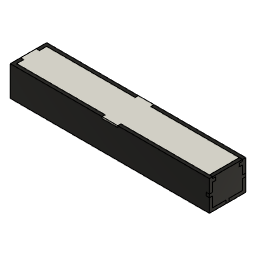
Soporte_LEDs v2 (Autodesk Fusion 360 design; units mm, degrees)
Autodesk Fusion 360 part; units mm, degrees
sketch "Boceto1" plane through (0, 0, 0) normal (0, 0, 1) x (1, 0, 0)
  line L0 (60, 8.75) -> (-60, 8.75)
  line L1 (-60, 8.75) -> (-60, -8.75)
  line L2 (-60, -8.75) -> (60, -8.75)
  line L3 (60, -8.75) -> (60, 8.75)
  line L4 (60, 8.75) -> (-60, -8.75) construction
  line L5 (-60, 8.75) -> (60, -8.75) construction
  dimension "d1" = 120
  dimension "d2" = 17.5
  constraint horizontal L0
  constraint perpendicular L0 L1
  constraint parallel L0 L2
  constraint parallel L1 L3
  constraint coincident L4 origin
  constraint coincident L5 origin
  measures "d1" distance of L1.end L2.end
  measures "d2" distance of L0.end L1.end
sketch "Boceto2" plane through (0, 0, 0) normal (0, 0, 1) x (1, 0, 0)
  line L0 (62, 9.5) -> (-62, 9.5)
  line L1 (-62, 9.5) -> (-62, -9.5)
  line L2 (-62, -9.5) -> (62, -9.5)
  line L3 (62, -9.5) -> (62, 9.5)
  line L4 (62, 9.5) -> (-62, -9.5) construction
  line L5 (-62, 9.5) -> (62, -9.5) construction
  line L6 (64, 11.5) -> (-64, 11.5)
  line L7 (-64, 11.5) -> (-64, -11.5)
  line L8 (-64, -11.5) -> (64, -11.5)
  line L9 (64, -11.5) -> (64, 11.5)
  line L10 (64, 11.5) -> (-64, -11.5) construction
  line L11 (-64, 11.5) -> (64, -11.5) construction
  dimension "d3" = 124
  dimension "d4" = 19
  dimension "d5" = 128
  dimension "d6" = 23
  constraint horizontal L0
  constraint perpendicular L0 L1
  constraint parallel L0 L2
  constraint parallel L1 L3
  constraint coincident L4 origin
  constraint coincident L5 origin
  constraint horizontal L6
  constraint perpendicular L6 L7
  constraint parallel L6 L8
  constraint parallel L7 L9
  constraint coincident L10 origin
  constraint coincident L11 origin
  measures "d3" distance of L1.end L2.end
  measures "d4" distance of L0.end L1.end
  measures "d5" distance of L7.end L8.end
  measures "d6" distance of L6.end L7.end
extrude "Extruir1" add sketch "Boceto2" along normal blind 2 contours L0 L1 L2 L3 makes body 1
extrude "Extruir2" add sketch "Boceto2" along normal blind 19 bodies 1
extrude "Extruir3" cut 1 faces at (64, -3.8333, 12.6667) along direction (-1, 0, 0) blind 2 on bodies 1 bodies 1
sketch "Boceto3" plane through (62, 0, 0) normal (1, 0, 0) x (0, 1, 0)
  line L0 (9.5, 19) -> (9.5, 2)
  line L1 (9.5, 2) -> (-9.5, 2)
  line L2 (-9.5, 2) -> (-9.5, 19)
  line L3 (-9.5, 19) -> (-11.5, 19)
  line L4 (-11.5, 19) -> (-11.5, 0)
  line L5 (-11.5, 0) -> (11.5, 0)
  line L6 (11.5, 0) -> (11.5, 19)
  line L7 (11.5, 19) -> (9.5, 19)
  line L8 (-11.5, 19) -> (11.5, 19)
  line L9 (11.5, 19) -> (11.5, 0)
  line L10 (11.5, 0) -> (-11.5, 0)
  line L11 (-11.5, 0) -> (-11.5, 19)
  line L12 (-11.5, 19) -> (-9.5, 19)
  line L13 (-9.5, 2) -> (9.5, 2)
  line L14 (9.5, 19) -> (11.5, 19)
  line L15 (-9.5, 19) -> (-9.5, 2)
  line L16 (9.5, 2) -> (9.5, 19)
  line L17 (-9.5, 7.5) -> (-7.5, 7.5)
  line L18 (-7.5, 7.5) -> (-7.5, 5.5)
  line L19 (-7.5, 5.5) -> (-9.5, 5.5)
  line L20 (-9.5, 5.5) -> (-9.5, 7.5)
  line L21 (0, 19) -> (0, 0) construction
  line L22 (-9.5, 18) -> (-7.5, 18)
  line L23 (-7.5, 18) -> (-7.5, 16)
  line L24 (-7.5, 16) -> (-9.5, 16)
  line L25 (-9.5, 16) -> (-9.5, 18)
  line L26 (9.5, 18) -> (7.5, 18)
  line L27 (7.5, 18) -> (7.5, 16)
  line L28 (7.5, 16) -> (9.5, 16)
  line L29 (9.5, 7.5) -> (7.5, 7.5)
  line L30 (7.5, 7.5) -> (7.5, 5.5)
  line L31 (7.5, 5.5) -> (9.5, 5.5)
  line L32 (-11.5, 9.5) -> (11.5, 9.5) construction
  line L33 (-9.5, 10.5) -> (-11.5, 10.5)
  line L34 (-11.5, 10.5) -> (-11.5, 8.5)
  line L35 (-11.5, 8.5) -> (-9.5, 8.5)
  line L36 (-9.5, 8.5) -> (-9.5, 10.5)
  line L37 (-9.5, 10.5) -> (-11.5, 8.5) construction
  line L38 (-11.5, 10.5) -> (-9.5, 8.5) construction
  line L39 (9.5, 10.5) -> (11.5, 10.5)
  line L40 (11.5, 10.5) -> (11.5, 8.5)
  line L41 (11.5, 8.5) -> (9.5, 8.5)
  line L42 (9.5, 8.5) -> (9.5, 10.5)
  line L43 (1, 2) -> (-1, 2)
  line L44 (-1, 2) -> (-1, 0)
  line L45 (-1, 0) -> (1, 0)
  line L46 (1, 0) -> (1, 2)
  line L47 (1, 2) -> (-1, 0) construction
  line L48 (-1, 2) -> (1, 0) construction
  point P0 (-10.5, 9.5)
  point P1 (0, 1)
  dimension "d13" = 2
  dimension "d14" = 2
  dimension "d15" = 3.5
  dimension "d16" = 2
  dimension "d17" = 2
  dimension "d18" = 1
  dimension "d30" = 2
  dimension "d31" = 2
  dimension "d32" = 2
  dimension "d33" = 2
  constraint horizontal L8
  constraint vertical L9
  constraint horizontal L10
  constraint vertical L11
  constraint coincident L5.end L6.start
  constraint coincident L3.end L4.start
  constraint coincident L2.end L3.start
  constraint coincident L1.end L2.start
  constraint coincident L0.end L1.start
  constraint coincident L0.start L7.end
  constraint coincident L6.end L7.start
  constraint horizontal L17
  constraint vertical L18
  constraint horizontal L19
  constraint vertical L20
  constraint coincident L2 L17.start
  constraint midpoint L8 L21.start
  constraint coincident L21.end origin
  constraint horizontal L22
  constraint vertical L23
  constraint horizontal L24
  constraint vertical L25
  constraint coincident L2 L22.start
  constraint symmetric L17.start L21 L29.start
  constraint symmetric L17.end L21 L29.end
  constraint symmetric L18.end L21 L30.end
  constraint symmetric L19.end L21 L31.end
  constraint symmetric L21 L22.start L26.start
  constraint symmetric L21 L22.end L26.end
  constraint symmetric L21 L23.end L27.end
  constraint symmetric L21 L24.end L28.end
  constraint midpoint L4 L32.start
  constraint midpoint L6 L32.end
  constraint horizontal L33
  constraint perpendicular L33 L34
  constraint parallel L33 L35
  constraint parallel L34 L36
  constraint coincident L37 P0
  constraint coincident L38 P0
  constraint coincident L32 P0
  constraint collinear L15 L36
  constraint symmetric L21 L33.start L39.start
  constraint symmetric L21 L33.end L39.end
  constraint symmetric L21 L34.end L40.end
  constraint symmetric L21 L35.end L41.end
  constraint horizontal L43
  constraint perpendicular L43 L44
  constraint parallel L43 L45
  constraint parallel L44 L46
  constraint coincident L47 P1
  constraint coincident L48 P1
  constraint coincident L21 P1
  constraint collinear L13 L43
  measures "d13" distance of L17.start L17.end
  measures "d14" distance of L17.start L19.end
  measures "d15" distance of L13 L19
  measures "d16" distance of L22.start L22.end
  measures "d17" distance of L22.start L24.end
  measures "d18" distance of L8 L22
  measures "d30" distance of L34.end L35.end
  measures "d31" distance of L33.end L34.end
  measures "d32" distance of L44.end L45.end
  measures "d33" distance of L43.end L44.end
extrude "Extruir4" add sketch "Boceto3" against normal blind 125 contours L0 L16 L26 L27 L28 | L2 L15 L22 L23 L24 L25 | L0 L16 L29 L30 L31 | L2 L15 L17 L18 L19 L20 bodies 1
sketch "Boceto4" plane through (-64, 0, 0) normal (-1, 0, 0) x (0, -1, 0)
  line L0 (-11.5, 0) -> (11.5, 0)
  line L1 (11.5, 0) -> (11.5, 19)
  line L2 (11.5, 19) -> (-11.5, 19)
  line L3 (-11.5, 19) -> (-11.5, 0)
  line L4 (-11.5, 19) -> (11.5, 19)
  line L5 (11.5, 19) -> (11.5, 0)
  line L6 (11.5, 0) -> (-11.5, 0)
  line L7 (-11.5, 0) -> (-11.5, 19)
  line L8 (-11.5, 19) -> (-9.5, 19)
  line L9 (-9.5, 19) -> (-9.5, 2)
  line L10 (-9.5, 0) -> (-11.5, 0)
  line L11 (-11.5, 0) -> (-11.5, 19)
  line L12 (-11.5, 0) -> (11.5, 0)
  line L13 (11.5, 0) -> (11.5, 2)
  line L14 (9.5, 2) -> (-9.5, 2)
  line L15 (-11.5, 2) -> (-11.5, 0)
  line L16 (11.5, 19) -> (9.5, 19)
  line L17 (9.5, 19) -> (9.5, 2)
  line L18 (9.5, 0) -> (11.5, 0)
  line L19 (11.5, 0) -> (11.5, 19)
  line L20 (-7, 11.5) -> (7, 11.5)
  line L21 (7, 11.5) -> (7, 7)
  line L22 (7, 7) -> (-7, 7)
  line L23 (-7, 7) -> (-7, 11.5)
  dimension "d21" = 2
  dimension "d22" = 2
  dimension "d23" = 2
  dimension "d24" = 14
  dimension "d25" = 4.5
  dimension "d26" = 2.5
  dimension "d27" = 5
  constraint horizontal L4
  constraint vertical L5
  constraint horizontal L6
  constraint vertical L7
  constraint coincident L0.end L1.start
  constraint coincident L2.end L3.start
  constraint horizontal L8
  constraint vertical L9
  constraint horizontal L10
  constraint vertical L11
  constraint horizontal L12
  constraint vertical L13
  constraint horizontal L14
  constraint vertical L15
  constraint coincident L5 L13.end
  constraint horizontal L16
  constraint vertical L17
  constraint horizontal L18
  constraint vertical L19
  constraint horizontal L20
  constraint vertical L21
  constraint horizontal L22
  constraint vertical L23
  measures "d21" distance of L2.end L8.end
  measures "d22" distance of L0.start L15.start
  measures "d23" distance of L1.end L16.end
  measures "d24" distance of L20.start L20.end
  measures "d25" distance of L20.start L22.end
  measures "d26" distance of L9 L23
  measures "d27" distance of L14 L22
extrude "Extruir5" cut sketch "Boceto4" against normal blind 2 contours L20 L21 L22 L23 bodies 1
extrude "Extruir6" cut sketch "Boceto3" against normal blind 2 contours L0 L6 L9 L16 L39 L40 L41 L42 | L2 L4 L11 L15 L33 L34 L35 L36 | L0 L16 L29 L30 L31 | L1 L5 L10 L13 L43 L44 L45 L46 | L2 L15 L17 L18 L19 L20 bodies 1
sketch "Boceto5" plane through (0, 0, 19) normal (0, 0, 1) x (-1, 0, 0)
  line L0 (-62, -9.5) -> (-62, -11.5)
  line L1 (-62, -11.5) -> (64, -11.5)
  line L2 (64, -11.5) -> (64, 11.5)
  line L3 (64, 11.5) -> (-62, 11.5)
  line L4 (-62, 11.5) -> (-62, 9.5)
  line L5 (-62, 9.5) -> (62, 9.5)
  line L6 (62, 9.5) -> (62, -9.5)
  line L7 (62, -9.5) -> (-62, -9.5)
  line L8 (-62, 0) -> (64, 0) construction
  line L9 (1, 11.5) -> (1, -11.5) construction
  line L10 (6, 9.5) -> (-4, 9.5)
  line L11 (-4, 9.5) -> (-4, 11.5)
  line L12 (-4, 11.5) -> (6, 11.5)
  line L13 (6, 11.5) -> (6, 9.5)
  line L14 (6, 9.5) -> (-4, 11.5) construction
  line L15 (-4, 9.5) -> (6, 11.5) construction
  line L16 (-4, -9.5) -> (-4, -11.5)
  line L17 (-4, -11.5) -> (6, -11.5)
  line L18 (6, -11.5) -> (6, -9.5)
  line L19 (6, -9.5) -> (-4, -9.5)
  line L20 (64, 5) -> (62, 5)
  line L21 (62, 5) -> (62, -5)
  line L22 (62, -5) -> (64, -5)
  line L23 (64, -5) -> (64, 5)
  line L24 (64, 5) -> (62, -5) construction
  line L25 (62, 5) -> (64, -5) construction
  line L26 (62, -9.5) -> (-60, -9.5)
  line L27 (-60, -9.5) -> (-60, 9.5)
  line L28 (-60, 9.5) -> (62, 9.5)
  line L29 (62, 9.5) -> (62, -9.5)
  line L30 (-62, 9.5) -> (-62, 1)
  point P0 (1, 10.5)
  point P1 (63, 0)
  dimension "d36" = 10
  dimension "d37" = 2
  dimension "d38" = 2
  dimension "d39" = 10
  dimension "d44" = 2
  constraint midpoint L2 L8.end
  constraint perpendicular L2 L8
  constraint midpoint L3 L9.start
  constraint midpoint L1 L9.end
  constraint horizontal L10
  constraint perpendicular L10 L11
  constraint parallel L10 L12
  constraint parallel L11 L13
  constraint coincident L14 P0
  constraint coincident L15 P0
  constraint coincident L9 P0
  constraint collinear L3 L12
  constraint symmetric L8 L10.start L18.end
  constraint symmetric L8 L10.end L16.start
  constraint symmetric L8 L11.end L16.end
  constraint symmetric L8 L12.end L17.end
  constraint horizontal L20
  constraint perpendicular L20 L21
  constraint parallel L20 L22
  constraint parallel L21 L23
  constraint coincident L24 P1
  constraint coincident L25 P1
  constraint coincident L8 P1
  constraint collinear L2 L23
  constraint horizontal L26
  constraint vertical L27
  constraint horizontal L28
  constraint vertical L29
  constraint coincident L5 L27.end
  constraint coincident L6.end L7.start
  measures "d36" distance of L11.end L12.end
  measures "d37" distance of L10.end L11.end
  measures "d38" distance of L21.end L22.end
  measures "d39" distance of L20.end L21.end
  measures "d44" distance of L27 L30
extrude "Extruir7" cut sketch "Boceto5" against normal blind 1 contours L1 L7 L16 L17 L18 L19 L26 | L3 L5 L10 L11 L12 L13 L28 | L2 L6 L20 L21 L22 L23 L29 bodies 1
extrude "Extruir8" add sketch "Boceto3" against normal blind 2 separate body contours L0 L1 L2 L8 L13 L15 L16 L17 L18 L19 L22 L23 L24 L26 L27 L28 L29 L30 L31 L36 L42 L43 | L0 L6 L9 L16 L39 L40 L41 L42 | L2 L4 L11 L15 L33 L34 L35 L36 | L0 L16 L29 L30 L31 | L1 L5 L10 L13 L43 L44 L45 L46 | L2 L15 L17 L18 L19 L20 makes body 2
extrude "Extruir9" add sketch "Boceto5" against normal blind 1 separate body contours L5 L6 L7 L10 L19 L21 L26 L27 L28 L29 | L1 L7 L16 L17 L18 L19 L26 | L3 L5 L10 L11 L12 L13 L28 | L2 L6 L20 L21 L22 L23 L29 makes body 3
named bodies: "Carcasa", "Tapa", "Acrilico"
